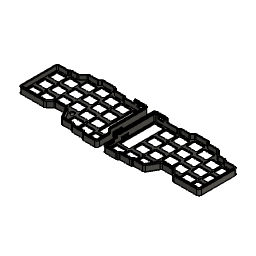
mriya-bumper-sla-v1.0.0 (Autodesk Fusion 360 design; units mm, degrees)
Autodesk Fusion 360 part; units mm, degrees
note: some values were not read from the file. Set by a fixed rule: which sketch regions a step uses.
(part 1 of 2)
sketch "mriya" plane through (0, 0, 0) normal (0, 0, 1) x (1, 0, 0)
  line L0 (-96.0213, 15.6719) -> (-89.7787, 21.9145) construction
  line L1 (-21.4858, 1.079) -> (-22.6142, 2.2074) construction
  line L2 (-133.1, 14.7932) -> (-98.1426, 14.7932) construction
  line L3 (-39.0716, 2.7932) -> (-24.0284, 2.7932) construction
  line L4 (-3.6, 0.4932) -> (-20.0716, 0.4932) construction
  line L5 (-59.4741, 6.1094) -> (-67.7517, 20.7608) construction
  line L6 (-40.4858, 3.379) -> (-41.6142, 4.5074) construction
  line L7 (-117.6142, 71.579) -> (-116.4858, 72.7074) construction
  line L8 (-96.0716, 81.2932) -> (-82.2284, 81.2932) construction
  line L9 (-133.1, 70.9932) -> (-119.0284, 70.9932) construction
  line L10 (-87.6574, 22.7932) -> (-71.2344, 22.7932) construction
  line L11 (-43.0284, 5.0932) -> (-57.7328, 5.0932) construction
  line L12 (-77.0716, 84.7932) -> (-59.7284, 84.7932) construction
  line L13 (-53.5716, 80.2932) -> (-40.7284, 80.2932) construction
  line L14 (-19.1, 19.4932) -> (-2.1, 19.4932) construction
  line L15 (-20.6, 20.9932) -> (-20.6, 77.9932) construction
  line L16 (-78.4858, 84.2074) -> (-80.8142, 81.879) construction
  line L17 (-58.3142, 84.2074) -> (-54.9858, 80.879) construction
  line L18 (-134.6, 69.4932) -> (-134.6, 16.2932) construction
  line L19 (-38.1858, 78.579) -> (-39.3142, 79.7074) construction
  line L20 (-94.4, 40.3932) -> (-94.4, 27.9932) construction
  line L21 (-93.6, 41.1932) -> (-81.2, 41.1932) construction
  line L22 (-93.6, 27.1932) -> (-81.2, 27.1932) construction
  line L23 (-80.4, 40.3932) -> (-80.4, 27.9932) construction
  line L24 (-37.4, 56.0932) -> (-37.4, 43.6932) construction
  line L25 (-36.6, 56.8932) -> (-24.2, 56.8932) construction
  line L26 (-36.6, 42.8932) -> (-24.2, 42.8932) construction
  line L27 (-23.4, 56.0932) -> (-23.4, 43.6932) construction
  line L28 (-56.4, 58.3932) -> (-56.4, 45.9932) construction
  line L29 (-55.6, 59.1932) -> (-43.2, 59.1932) construction
  line L30 (-55.6, 45.1932) -> (-43.2, 45.1932) construction
  line L31 (-42.4, 58.3932) -> (-42.4, 45.9932) construction
  line L32 (-132.4, 68.0932) -> (-132.4, 55.6932) construction
  line L33 (-131.6, 68.8932) -> (-119.2, 68.8932) construction
  line L34 (-131.6, 54.8932) -> (-119.2, 54.8932) construction
  line L35 (-118.4, 68.0932) -> (-118.4, 55.6932) construction
  line L36 (-56.4, 39.3932) -> (-56.4, 26.9932) construction
  line L37 (-55.6, 40.1932) -> (-43.2, 40.1932) construction
  line L38 (-55.6, 26.1932) -> (-43.2, 26.1932) construction
  line L39 (-42.4, 39.3932) -> (-42.4, 26.9932) construction
  line L40 (-37.4, 18.0932) -> (-37.4, 5.6932) construction
  line L41 (-36.6, 18.8932) -> (-24.2, 18.8932) construction
  line L42 (-36.6, 4.8932) -> (-24.2, 4.8932) construction
  line L43 (-23.4, 18.0932) -> (-23.4, 5.6932) construction
  line L44 (-18.4, 15.7932) -> (-18.4, 3.3932) construction
  line L45 (-17.6, 16.5932) -> (-5.2, 16.5932) construction
  line L46 (-17.6, 2.5932) -> (-5.2, 2.5932) construction
  line L47 (-4.4, 15.7932) -> (-4.4, 3.3932) construction
  line L48 (-132.4, 49.0932) -> (-132.4, 36.6932) construction
  line L49 (-131.6, 49.8932) -> (-119.2, 49.8932) construction
  line L50 (-131.6, 35.8932) -> (-119.2, 35.8932) construction
  line L51 (-118.4, 49.0932) -> (-118.4, 36.6932) construction
  line L52 (-113.4, 51.3932) -> (-113.4, 38.9932) construction
  line L53 (-112.6, 52.1932) -> (-100.2, 52.1932) construction
  line L54 (-112.6, 38.1932) -> (-100.2, 38.1932) construction
  line L55 (-99.4, 51.3932) -> (-99.4, 38.9932) construction
  line L56 (-132.4, 30.0932) -> (-132.4, 17.6932) construction
  line L57 (-131.6, 30.8932) -> (-119.2, 30.8932) construction
  line L58 (-131.6, 16.8932) -> (-119.2, 16.8932) construction
  line L59 (-118.4, 30.0932) -> (-118.4, 17.6932) construction
  line L60 (-56.4, 20.3932) -> (-56.4, 7.9932) construction
  line L61 (-55.6, 21.1932) -> (-43.2, 21.1932) construction
  line L62 (-55.6, 7.1932) -> (-43.2, 7.1932) construction
  line L63 (-42.4, 20.3932) -> (-42.4, 7.9932) construction
  line L64 (-75.4, 43.8932) -> (-75.4, 31.4932) construction
  line L65 (-74.6, 44.6932) -> (-62.2, 44.6932) construction
  line L66 (-74.6, 30.6932) -> (-62.2, 30.6932) construction
  line L67 (-61.4, 43.8932) -> (-61.4, 31.4932) construction
  line L68 (-75.4, 81.8932) -> (-75.4, 69.4932) construction
  line L69 (-74.6, 82.6932) -> (-62.2, 82.6932) construction
  line L70 (-74.6, 68.6932) -> (-62.2, 68.6932) construction
  line L71 (-61.4, 81.8932) -> (-61.4, 69.4932) construction
  line L72 (-37.4, 37.0932) -> (-37.4, 24.6932) construction
  line L73 (-36.6, 37.8932) -> (-24.2, 37.8932) construction
  line L74 (-36.6, 23.8932) -> (-24.2, 23.8932) construction
  line L75 (-23.4, 37.0932) -> (-23.4, 24.6932) construction
  line L76 (-113.4, 32.3932) -> (-113.4, 19.9932) construction
  line L77 (-112.6, 33.1932) -> (-100.2, 33.1932) construction
  line L78 (-112.6, 19.1932) -> (-100.2, 19.1932) construction
  line L79 (-99.4, 32.3932) -> (-99.4, 19.9932) construction
  line L80 (-56.4, 77.3932) -> (-56.4, 64.9932) construction
  line L81 (-55.6, 78.1932) -> (-43.2, 78.1932) construction
  line L82 (-55.6, 64.1932) -> (-43.2, 64.1932) construction
  line L83 (-42.4, 77.3932) -> (-42.4, 64.9932) construction
  line L84 (-37.4, 75.0932) -> (-37.4, 62.6932) construction
  line L85 (-36.6, 75.8932) -> (-24.2, 75.8932) construction
  line L86 (-36.6, 61.8932) -> (-24.2, 61.8932) construction
  line L87 (-23.4, 75.0932) -> (-23.4, 62.6932) construction
  line L88 (-113.4, 70.3932) -> (-113.4, 57.9932) construction
  line L89 (-112.6, 71.1932) -> (-100.2, 71.1932) construction
  line L90 (-112.6, 57.1932) -> (-100.2, 57.1932) construction
  line L91 (-99.4, 70.3932) -> (-99.4, 57.9932) construction
  line L92 (-94.4, 59.3932) -> (-94.4, 46.9932) construction
  line L93 (-93.6, 60.1932) -> (-81.2, 60.1932) construction
  line L94 (-93.6, 46.1932) -> (-81.2, 46.1932) construction
  line L95 (-80.4, 59.3932) -> (-80.4, 46.9932) construction
  line L96 (-75.4, 62.8932) -> (-75.4, 50.4932) construction
  line L97 (-74.6, 63.6932) -> (-62.2, 63.6932) construction
  line L98 (-74.6, 49.6932) -> (-62.2, 49.6932) construction
  line L99 (-61.4, 62.8932) -> (-61.4, 50.4932) construction
  line L100 (-94.4, 78.3932) -> (-94.4, 65.9932) construction
  line L101 (-93.6, 79.1932) -> (-81.2, 79.1932) construction
  line L102 (-93.6, 65.1932) -> (-81.2, 65.1932) construction
  line L103 (-80.4, 78.3932) -> (-80.4, 65.9932) construction
  circle A0 centre (-115.9, 53.5432) radius 1.6
  circle A1 centre (-115.9, 34.5432) radius 1.6
  circle A2 centre (-63.5, 23.5932) radius 3.5
  circle A3 centre (-39.9, 22.5432) radius 1.6
  circle A4 centre (-39.9, 60.5432) radius 1.6
  arc A5 (-38.1858, 78.579) -> (-36.7716, 77.9932) centre (-36.7716, 79.9932) ccw construction
  arc A6 (-39.3142, 79.7074) -> (-40.7284, 80.2932) centre (-40.7285, 78.2931) ccw construction
  arc A7 (-54.9858, 80.879) -> (-53.5716, 80.2932) centre (-53.5716, 82.2931) ccw construction
  arc A8 (-58.3142, 84.2074) -> (-59.7284, 84.7932) centre (-59.7285, 82.7931) ccw construction
  arc A9 (-77.0716, 84.7932) -> (-78.4858, 84.2074) centre (-77.0716, 82.7933) ccw construction
  arc A10 (-82.2284, 81.2932) -> (-80.8142, 81.879) centre (-82.2284, 83.2932) ccw construction
  arc A11 (-96.0716, 81.2932) -> (-97.4858, 80.7074) centre (-96.0716, 79.2933) ccw construction
  arc A12 (-115.0716, 73.2932) -> (-116.4858, 72.7074) centre (-115.0716, 71.2933) ccw construction
  arc A13 (-119.0284, 70.9932) -> (-117.6142, 71.579) centre (-119.0284, 72.9932) ccw construction
  arc A14 (-133.1, 70.9932) -> (-134.6, 69.4932) centre (-133.1, 69.4932) ccw construction
  arc A15 (-134.6, 16.2932) -> (-133.1, 14.7932) centre (-133.1, 16.2932) ccw construction
  arc A16 (-98.1426, 14.7932) -> (-96.0213, 15.6719) centre (-98.1426, 17.7931) ccw construction
  arc A17 (-87.6574, 22.7932) -> (-89.7787, 21.9145) centre (-87.6573, 19.7931) ccw construction
  arc A18 (-67.7517, 20.7608) -> (-71.2344, 22.7932) centre (-71.2344, 18.793) ccw construction
  arc A19 (-59.4741, 6.1094) -> (-57.7328, 5.0932) centre (-57.7328, 7.0932) ccw construction
  arc A20 (-41.6142, 4.5074) -> (-43.0284, 5.0932) centre (-43.0284, 3.0933) ccw construction
  arc A21 (-40.4858, 3.379) -> (-39.0716, 2.7932) centre (-39.0715, 4.7933) ccw construction
  arc A22 (-22.6142, 2.2074) -> (-24.0284, 2.7932) centre (-24.0284, 0.7933) ccw construction
  arc A23 (-21.4858, 1.079) -> (-20.0716, 0.4932) centre (-20.0715, 2.4933) ccw construction
  arc A24 (-3.6, 0.4932) -> (-2.1, 1.9932) centre (-3.6, 1.9932) ccw construction
  arc A25 (-20.6, 20.9932) -> (-19.1, 19.4932) centre (-19.1, 20.9932) ccw construction
  line L104 (-2.1, 1.9932) -> (-2.1, 76.4932) construction
  line L105 (-36.7716, 77.9932) -> (-3.6, 77.9932) construction
  arc A26 (-2.1, 76.4932) -> (-3.6, 77.9932) centre (-3.6, 76.4932) ccw construction
  arc A27 (-131.6, 68.8932) -> (-132.4, 68.0932) centre (-131.6, 68.0932) ccw construction
  arc A28 (-118.4, 68.0932) -> (-119.2, 68.8932) centre (-119.2, 68.0932) ccw construction
  arc A29 (-119.2, 54.8932) -> (-118.4, 55.6932) centre (-119.2, 55.6932) ccw construction
  arc A30 (-132.4, 55.6932) -> (-131.6, 54.8932) centre (-131.6, 55.6932) ccw construction
  arc A31 (-131.6, 49.8932) -> (-132.4, 49.0932) centre (-131.6, 49.0932) ccw construction
  arc A32 (-118.4, 49.0932) -> (-119.2, 49.8932) centre (-119.2, 49.0932) ccw construction
  arc A33 (-119.2, 35.8932) -> (-118.4, 36.6932) centre (-119.2, 36.6932) ccw construction
  arc A34 (-132.4, 36.6932) -> (-131.6, 35.8932) centre (-131.6, 36.6932) ccw construction
  arc A35 (-131.6, 30.8932) -> (-132.4, 30.0932) centre (-131.6, 30.0932) ccw construction
  arc A36 (-118.4, 30.0932) -> (-119.2, 30.8932) centre (-119.2, 30.0932) ccw construction
  arc A37 (-119.2, 16.8932) -> (-118.4, 17.6932) centre (-119.2, 17.6932) ccw construction
  arc A38 (-132.4, 17.6932) -> (-131.6, 16.8932) centre (-131.6, 17.6932) ccw construction
  arc A39 (-113.4, 19.9932) -> (-112.6, 19.1932) centre (-112.6, 19.9932) ccw construction
  arc A40 (-100.2, 19.1932) -> (-99.4, 19.9932) centre (-100.2, 19.9932) ccw construction
  arc A41 (-99.4, 32.3932) -> (-100.2, 33.1932) centre (-100.2, 32.3932) ccw construction
  arc A42 (-112.6, 33.1932) -> (-113.4, 32.3932) centre (-112.6, 32.3932) ccw construction
  arc A43 (-100.2, 38.1932) -> (-99.4, 38.9932) centre (-100.2, 38.9932) ccw construction
  arc A44 (-113.4, 38.9932) -> (-112.6, 38.1932) centre (-112.6, 38.9932) ccw construction
  arc A45 (-112.6, 52.1932) -> (-113.4, 51.3932) centre (-112.6, 51.3932) ccw construction
  arc A46 (-99.4, 51.3932) -> (-100.2, 52.1932) centre (-100.2, 51.3932) ccw construction
  arc A47 (-113.4, 57.9932) -> (-112.6, 57.1932) centre (-112.6, 57.9932) ccw construction
  arc A48 (-100.2, 57.1932) -> (-99.4, 57.9932) centre (-100.2, 57.9932) ccw construction
  arc A49 (-99.4, 70.3932) -> (-100.2, 71.1932) centre (-100.2, 70.3932) ccw construction
  arc A50 (-112.6, 71.1932) -> (-113.4, 70.3932) centre (-112.6, 70.3932) ccw construction
  arc A51 (-93.6, 79.1932) -> (-94.4, 78.3932) centre (-93.6, 78.3932) ccw construction
  arc A52 (-80.4, 78.3932) -> (-81.2, 79.1932) centre (-81.2, 78.3932) ccw construction
  arc A53 (-81.2, 65.1932) -> (-80.4, 65.9932) centre (-81.2, 65.9932) ccw construction
  arc A54 (-94.4, 65.9932) -> (-93.6, 65.1932) centre (-93.6, 65.9932) ccw construction
  arc A55 (-93.6, 60.1932) -> (-94.4, 59.3932) centre (-93.6, 59.3932) ccw construction
  arc A56 (-80.4, 59.3932) -> (-81.2, 60.1932) centre (-81.2, 59.3932) ccw construction
  arc A57 (-81.2, 46.1932) -> (-80.4, 46.9932) centre (-81.2, 46.9932) ccw construction
  arc A58 (-94.4, 46.9932) -> (-93.6, 46.1932) centre (-93.6, 46.9932) ccw construction
  arc A59 (-93.6, 41.1932) -> (-94.4, 40.3932) centre (-93.6, 40.3932) ccw construction
  arc A60 (-94.4, 27.9932) -> (-93.6, 27.1932) centre (-93.6, 27.9932) ccw construction
  arc A61 (-81.2, 27.1932) -> (-80.4, 27.9932) centre (-81.2, 27.9932) ccw construction
  arc A62 (-80.4, 40.3932) -> (-81.2, 41.1932) centre (-81.2, 40.3932) ccw construction
  arc A63 (-75.4, 31.4932) -> (-74.6, 30.6932) centre (-74.6, 31.4932) ccw construction
  arc A64 (-74.6, 44.6932) -> (-75.4, 43.8932) centre (-74.6, 43.8932) ccw construction
  arc A65 (-61.4, 43.8932) -> (-62.2, 44.6932) centre (-62.2, 43.8932) ccw construction
  arc A66 (-62.2, 30.6932) -> (-61.4, 31.4932) centre (-62.2, 31.4932) ccw construction
  arc A67 (-62.2, 49.6932) -> (-61.4, 50.4932) centre (-62.2, 50.4932) ccw construction
  arc A68 (-75.4, 50.4932) -> (-74.6, 49.6932) centre (-74.6, 50.4932) ccw construction
  arc A69 (-74.6, 63.6932) -> (-75.4, 62.8932) centre (-74.6, 62.8932) ccw construction
  arc A70 (-61.4, 62.8932) -> (-62.2, 63.6932) centre (-62.2, 62.8932) ccw construction
  arc A71 (-62.2, 68.6932) -> (-61.4, 69.4932) centre (-62.2, 69.4932) ccw construction
  arc A72 (-75.4, 69.4932) -> (-74.6, 68.6932) centre (-74.6, 69.4932) ccw construction
  arc A73 (-74.6, 82.6932) -> (-75.4, 81.8932) centre (-74.6, 81.8932) ccw construction
  arc A74 (-61.4, 81.8932) -> (-62.2, 82.6932) centre (-62.2, 81.8932) ccw construction
  arc A75 (-55.6, 78.1932) -> (-56.4, 77.3932) centre (-55.6, 77.3932) ccw construction
  arc A76 (-56.4, 64.9932) -> (-55.6, 64.1932) centre (-55.6, 64.9932) ccw construction
  arc A77 (-43.2, 64.1932) -> (-42.4, 64.9932) centre (-43.2, 64.9932) ccw construction
  arc A78 (-42.4, 77.3932) -> (-43.2, 78.1932) centre (-43.2, 77.3932) ccw construction
  arc A79 (-42.4, 58.3932) -> (-43.2, 59.1932) centre (-43.2, 58.3932) ccw construction
  arc A80 (-55.6, 59.1932) -> (-56.4, 58.3932) centre (-55.6, 58.3932) ccw construction
  arc A81 (-56.4, 45.9932) -> (-55.6, 45.1932) centre (-55.6, 45.9932) ccw construction
  arc A82 (-43.2, 45.1932) -> (-42.4, 45.9932) centre (-43.2, 45.9932) ccw construction
  arc A83 (-42.4, 39.3932) -> (-43.2, 40.1932) centre (-43.2, 39.3932) ccw construction
  arc A84 (-55.6, 40.1932) -> (-56.4, 39.3932) centre (-55.6, 39.3932) ccw construction
  arc A85 (-56.4, 26.9932) -> (-55.6, 26.1932) centre (-55.6, 26.9932) ccw construction
  arc A86 (-43.2, 26.1932) -> (-42.4, 26.9932) centre (-43.2, 26.9932) ccw construction
  arc A87 (-42.4, 20.3932) -> (-43.2, 21.1932) centre (-43.2, 20.3932) ccw construction
  arc A88 (-55.6, 21.1932) -> (-56.4, 20.3932) centre (-55.6, 20.3932) ccw construction
  arc A89 (-56.4, 7.9932) -> (-55.6, 7.1932) centre (-55.6, 7.9932) ccw construction
  arc A90 (-43.2, 7.1932) -> (-42.4, 7.9932) centre (-43.2, 7.9932) ccw construction
  arc A91 (-37.4, 5.6932) -> (-36.6, 4.8932) centre (-36.6, 5.6932) ccw construction
  arc A92 (-24.2, 4.8932) -> (-23.4, 5.6932) centre (-24.2, 5.6932) ccw construction
  arc A93 (-23.4, 18.0932) -> (-24.2, 18.8932) centre (-24.2, 18.0932) ccw construction
  arc A94 (-36.6, 18.8932) -> (-37.4, 18.0932) centre (-36.6, 18.0932) ccw construction
  arc A95 (-18.4, 3.3932) -> (-17.6, 2.5932) centre (-17.6, 3.3932) ccw construction
  arc A96 (-5.2, 2.5932) -> (-4.4, 3.3932) centre (-5.2, 3.3932) ccw construction
  arc A97 (-4.4, 15.7932) -> (-5.2, 16.5932) centre (-5.2, 15.7932) ccw construction
  arc A98 (-17.6, 16.5932) -> (-18.4, 15.7932) centre (-17.6, 15.7932) ccw construction
  arc A99 (-24.2, 23.8932) -> (-23.4, 24.6932) centre (-24.2, 24.6932) ccw construction
  arc A100 (-37.4, 24.6932) -> (-36.6, 23.8932) centre (-36.6, 24.6932) ccw construction
  arc A101 (-36.6, 37.8932) -> (-37.4, 37.0932) centre (-36.6, 37.0932) ccw construction
  arc A102 (-23.4, 37.0932) -> (-24.2, 37.8932) centre (-24.2, 37.0932) ccw construction
  arc A103 (-24.2, 42.8932) -> (-23.4, 43.6932) centre (-24.2, 43.6932) ccw construction
  arc A104 (-37.4, 43.6932) -> (-36.6, 42.8932) centre (-36.6, 43.6932) ccw construction
  arc A105 (-36.6, 56.8932) -> (-37.4, 56.0932) centre (-36.6, 56.0932) ccw construction
  arc A106 (-23.4, 56.0932) -> (-24.2, 56.8932) centre (-24.2, 56.0932) ccw construction
  arc A107 (-24.2, 61.8932) -> (-23.4, 62.6932) centre (-24.2, 62.6932) ccw construction
  arc A108 (-37.4, 62.6932) -> (-36.6, 61.8932) centre (-36.6, 62.6932) ccw construction
  arc A109 (-36.6, 75.8932) -> (-37.4, 75.0932) centre (-36.6, 75.0932) ccw construction
  arc A110 (-23.4, 75.0932) -> (-24.2, 75.8932) centre (-24.2, 75.0932) ccw construction
  line L106 (-117.6496, 71.6144) -> (-116.5212, 72.7428)
  arc A111 (-115.0716, 73.3432) -> (-116.5212, 72.7428) centre (-115.0716, 71.2933) ccw
  arc A112 (-96.0716, 81.3432) -> (-97.5212, 80.7428) centre (-96.0716, 79.2933) ccw
  line L107 (-96.0716, 81.3432) -> (-82.2284, 81.3432)
  arc A113 (-82.2284, 81.3432) -> (-80.8496, 81.9144) centre (-82.2284, 83.2932) ccw
  line L108 (-78.5212, 84.2428) -> (-80.8496, 81.9144)
  arc A114 (-77.0716, 84.8432) -> (-78.5212, 84.2428) centre (-77.0716, 82.7933) ccw
  line L109 (-77.0716, 84.8432) -> (-59.7284, 84.8432)
  arc A115 (-58.2788, 84.2427) -> (-59.7284, 84.8432) centre (-59.7285, 82.7931) ccw
  line L110 (-58.2788, 84.2427) -> (-54.9504, 80.9144)
  arc A116 (-54.9504, 80.9144) -> (-53.5716, 80.3432) centre (-53.5716, 82.2931) ccw
  line L111 (-53.5716, 80.3432) -> (-40.7284, 80.3432)
  arc A117 (-39.2788, 79.7427) -> (-40.7284, 80.3432) centre (-40.7285, 78.2931) ccw
  line L112 (-38.1504, 78.6144) -> (-39.2788, 79.7427)
  arc A118 (-38.1504, 78.6144) -> (-36.7716, 78.0432) centre (-36.7716, 79.9932) ccw
  line L113 (-36.7716, 78.0432) -> (-3.6, 78.0432)
  arc A119 (-2.05, 76.4932) -> (-3.6, 78.0432) centre (-3.6, 76.4932) ccw
  line L114 (-2.05, 1.9932) -> (-2.05, 76.4932)
  arc A120 (-3.6, 0.4432) -> (-2.05, 1.9932) centre (-3.6, 1.9932) ccw
  line L115 (-3.6, 0.4432) -> (-20.0716, 0.4432)
  arc A121 (-21.5212, 1.0437) -> (-20.0716, 0.4432) centre (-20.0715, 2.4933) ccw
  line L116 (-21.5212, 1.0437) -> (-22.6496, 2.172)
  arc A122 (-22.6496, 2.172) -> (-24.0284, 2.7432) centre (-24.0284, 0.7933) ccw
  line L117 (-39.0716, 2.7432) -> (-24.0284, 2.7432)
  arc A123 (-40.5212, 3.3437) -> (-39.0716, 2.7432) centre (-39.0715, 4.7933) ccw
  line L118 (-40.5212, 3.3437) -> (-41.6496, 4.472)
  arc A124 (-41.6496, 4.472) -> (-43.0284, 5.0432) centre (-43.0284, 3.0933) ccw
  line L119 (-43.0284, 5.0432) -> (-57.7328, 5.0432)
  arc A125 (-59.5176, 6.0848) -> (-57.7328, 5.0432) centre (-57.7328, 7.0932) ccw
  line L120 (-59.5176, 6.0848) -> (-67.7952, 20.7362)
  arc A126 (-67.7952, 20.7362) -> (-71.2344, 22.7432) centre (-71.2344, 18.793) ccw
  line L121 (-87.6574, 22.7432) -> (-71.2344, 22.7432)
  arc A127 (-87.6574, 22.7432) -> (-89.7433, 21.8791) centre (-87.6573, 19.7931) ccw
  line L122 (-95.9859, 15.6365) -> (-89.7433, 21.8791)
  arc A128 (-98.1426, 14.7432) -> (-95.9859, 15.6365) centre (-98.1426, 17.7931) ccw
  line L123 (-133.1, 14.7432) -> (-98.1426, 14.7432)
  arc A129 (-134.65, 16.2932) -> (-133.1, 14.7432) centre (-133.1, 16.2932) ccw
  line L124 (-134.65, 69.4932) -> (-134.65, 16.2932)
  arc A130 (-133.1, 71.0432) -> (-134.65, 69.4932) centre (-133.1, 69.4932) ccw
  line L125 (-133.1, 71.0432) -> (-119.0284, 71.0432)
  arc A131 (-119.0284, 71.0432) -> (-117.6496, 71.6144) centre (-119.0284, 72.9932) ccw
  line L126 (-77.7136, 87.3432) -> (-59.0864, 87.3432)
  arc A132 (0.45, 76.4932) -> (-3.6, 80.5432) centre (-3.6, 76.4932) ccw
  line L127 (0.45, 1.9932) -> (0.45, 76.4932)
  arc A133 (-3.6, -2.0568) -> (0.45, 1.9932) centre (-3.6, 1.9932) ccw
  line L128 (-3.6, -2.0568) -> (-20.7136, -2.0568)
  line L129 (-133.1, 12.2432) -> (-97.7077, 12.2432)
  arc A134 (-137.15, 16.2932) -> (-133.1, 12.2432) centre (-133.1, 16.2932) ccw
  line L130 (-137.15, 69.4932) -> (-137.15, 16.2932)
  arc A135 (-133.1, 73.5432) -> (-137.15, 69.4932) centre (-133.1, 69.4932) ccw
  circle A136 centre (-17.6, 22.4932) radius 1.1 construction
  circle A137 centre (-5.2, 22.4932) radius 1.1 construction
  line L131 (-2.05, 19.1932) -> (0.45, 19.1932)
  line L132 (-20.9, 78.0432) -> (-20.9, 80.5432)
  line L133 (-19.7, 77.8432) -> (-19.7, 78.0432)
  line L134 (-19.1, 77.2432) -> (-3.65, 77.2432)
  line L135 (-2.25, 21.1932) -> (-2.05, 21.1932)
  line L136 (-2.85, 21.7932) -> (-2.85, 76.4432)
  arc A138 (-2.85, 76.4432) -> (-3.65, 77.2432) centre (-3.65, 76.4432) ccw
  arc A139 (-19.7, 77.8432) -> (-19.1, 77.2432) centre (-19.1, 77.8432) ccw
  arc A140 (-2.85, 21.7932) -> (-2.25, 21.1932) centre (-2.25, 21.7932) ccw
  line L137 (-2.05, 14.5932) -> (-2.25, 14.5932)
  line L138 (-2.85, 13.9932) -> (-2.85, 5.1932)
  line L139 (-2.25, 4.5932) -> (-2.05, 4.5932)
  arc A141 (-2.25, 14.5932) -> (-2.85, 13.9932) centre (-2.25, 13.9932) ccw
  arc A142 (-2.85, 5.1932) -> (-2.25, 4.5932) centre (-2.25, 5.1932) ccw
  line L140 (-97.4858, 80.7074) -> (-104.0213, 74.1719) construction
  line L141 (-115.0716, 73.2932) -> (-106.1426, 73.2932) construction
  line L142 (-97.5212, 80.7428) -> (-104.0567, 74.2072)
  line L143 (-106.1426, 73.3432) -> (-115.0716, 73.3432)
  arc A143 (-106.1426, 73.3432) -> (-104.0567, 74.2072) centre (-106.1426, 76.2932) ccw
  arc A144 (-106.1426, 73.2932) -> (-104.0213, 74.1719) centre (-106.1426, 76.2932) ccw construction
  line L144 (-87.0153, 20.2432) -> (-72.1389, 20.2432)
  arc A145 (-87.0153, 20.2432) -> (-88.4295, 19.6574) centre (-87.0153, 18.2432) ccw
  arc A146 (-69.5269, 18.7189) -> (-72.1389, 20.2432) centre (-72.1389, 17.2432) ccw
  line L145 (-106.3705, 75.8432) -> (-115.7136, 75.8432)
  line L146 (-133.1, 73.5432) -> (-119.6705, 73.5432)
  line L147 (-96.7136, 83.8432) -> (-82.8705, 83.8432)
  line L148 (-52.9295, 82.8432) -> (-40.0864, 82.8432)
  line L149 (-36.1295, 80.5432) -> (-3.6, 80.5432)
  line L150 (-39.7136, 0.2432) -> (-24.6705, 0.2432)
  line L151 (-58.3456, 2.5432) -> (-43.6705, 2.5432)
  arc A147 (-59.7284, 82.7932) -> (-59.7285, 82.7932) centre (-59.7285, 82.7931) ccw
  arc A148 (-40.7284, 78.2932) -> (-40.7285, 78.2932) centre (-40.7285, 78.2931) ccw
  arc A149 (-20.0716, 2.4932) -> (-20.0715, 2.4932) centre (-20.0715, 2.4933) ccw
  arc A150 (-39.0716, 4.7932) -> (-39.0715, 4.7932) centre (-39.0715, 4.7933) ccw
  line L152 (-118.9, 54.8932) -> (-131.9, 54.8932)
  line L153 (-133.9, 56.8932) -> (-133.9, 66.8932)
  line L154 (-131.9, 68.8932) -> (-118.9, 68.8932)
  line L155 (-116.9, 66.8932) -> (-116.9, 56.8932)
  arc A151 (-116.9, 66.8932) -> (-118.9, 68.8932) centre (-118.9, 66.8932) ccw
  arc A152 (-118.9, 54.8932) -> (-116.9, 56.8932) centre (-118.9, 56.8932) ccw
  arc A153 (-133.9, 56.8932) -> (-131.9, 54.8932) centre (-131.9, 56.8932) ccw
  arc A154 (-131.9, 68.8932) -> (-133.9, 66.8932) centre (-131.9, 66.8932) ccw
  arc A155 (-118.9, 35.8932) -> (-116.9, 37.8932) centre (-118.9, 37.8932) ccw
  line L156 (-118.9, 35.8932) -> (-131.9, 35.8932)
  arc A156 (-133.9, 37.8932) -> (-131.9, 35.8932) centre (-131.9, 37.8932) ccw
  line L157 (-133.9, 37.8932) -> (-133.9, 47.8932)
  arc A157 (-131.9, 49.8932) -> (-133.9, 47.8932) centre (-131.9, 47.8932) ccw
  line L158 (-131.9, 49.8932) -> (-118.9, 49.8932)
  arc A158 (-116.9, 47.8932) -> (-118.9, 49.8932) centre (-118.9, 47.8932) ccw
  line L159 (-116.9, 47.8932) -> (-116.9, 37.8932)
  arc A159 (-118.9, 16.8932) -> (-116.9, 18.8932) centre (-118.9, 18.8932) ccw
  line L160 (-118.9, 16.8932) -> (-131.9, 16.8932)
  arc A160 (-133.9, 18.8932) -> (-131.9, 16.8932) centre (-131.9, 18.8932) ccw
  line L161 (-133.9, 18.8932) -> (-133.9, 28.8932)
  arc A161 (-131.9, 30.8932) -> (-133.9, 28.8932) centre (-131.9, 28.8932) ccw
  line L162 (-131.9, 30.8932) -> (-118.9, 30.8932)
  arc A162 (-116.9, 28.8932) -> (-118.9, 30.8932) centre (-118.9, 28.8932) ccw
  line L163 (-116.9, 28.8932) -> (-116.9, 18.8932)
  arc A163 (-99.9, 57.1932) -> (-97.9, 59.1932) centre (-99.9, 59.1932) ccw
  line L164 (-99.9, 57.1932) -> (-112.9, 57.1932)
  arc A164 (-114.9, 59.1932) -> (-112.9, 57.1932) centre (-112.9, 59.1932) ccw
  line L165 (-114.9, 59.1932) -> (-114.9, 69.1932)
  arc A165 (-112.9, 71.1932) -> (-114.9, 69.1932) centre (-112.9, 69.1932) ccw
  line L166 (-112.9, 71.1932) -> (-99.9, 71.1932)
  arc A166 (-97.9, 69.1932) -> (-99.9, 71.1932) centre (-99.9, 69.1932) ccw
  line L167 (-97.9, 69.1932) -> (-97.9, 59.1932)
  arc A167 (-99.9, 38.1932) -> (-97.9, 40.1932) centre (-99.9, 40.1932) ccw
  line L168 (-99.9, 38.1932) -> (-112.9, 38.1932)
  arc A168 (-114.9, 40.1932) -> (-112.9, 38.1932) centre (-112.9, 40.1932) ccw
  line L169 (-114.9, 40.1932) -> (-114.9, 50.1932)
  arc A169 (-112.9, 52.1932) -> (-114.9, 50.1932) centre (-112.9, 50.1932) ccw
  line L170 (-112.9, 52.1932) -> (-99.9, 52.1932)
  arc A170 (-97.9, 50.1932) -> (-99.9, 52.1932) centre (-99.9, 50.1932) ccw
  line L171 (-97.9, 50.1932) -> (-97.9, 40.1932)
  arc A171 (-99.9, 19.1932) -> (-97.9, 21.1932) centre (-99.9, 21.1932) ccw
  line L172 (-99.9, 19.1932) -> (-112.9, 19.1932)
  arc A172 (-114.9, 21.1932) -> (-112.9, 19.1932) centre (-112.9, 21.1932) ccw
  line L173 (-114.9, 21.1932) -> (-114.9, 31.1932)
  arc A173 (-112.9, 33.1932) -> (-114.9, 31.1932) centre (-112.9, 31.1932) ccw
  line L174 (-112.9, 33.1932) -> (-99.9, 33.1932)
  arc A174 (-97.9, 31.1932) -> (-99.9, 33.1932) centre (-99.9, 31.1932) ccw
  line L175 (-97.9, 31.1932) -> (-97.9, 21.1932)
  arc A175 (-80.9, 65.1932) -> (-78.9, 67.1932) centre (-80.9, 67.1932) ccw
  line L176 (-80.9, 65.1932) -> (-93.9, 65.1932)
  arc A176 (-95.9, 67.1932) -> (-93.9, 65.1932) centre (-93.9, 67.1932) ccw
  line L177 (-95.9, 67.1932) -> (-95.9, 77.1932)
  arc A177 (-93.9, 79.1932) -> (-95.9, 77.1932) centre (-93.9, 77.1932) ccw
  line L178 (-93.9, 79.1932) -> (-80.9, 79.1932)
  arc A178 (-78.9, 77.1932) -> (-80.9, 79.1932) centre (-80.9, 77.1932) ccw
  line L179 (-78.9, 77.1932) -> (-78.9, 67.1932)
  arc A179 (-80.9, 46.1932) -> (-78.9, 48.1932) centre (-80.9, 48.1932) ccw
  line L180 (-80.9, 46.1932) -> (-93.9, 46.1932)
  arc A180 (-95.9, 48.1932) -> (-93.9, 46.1932) centre (-93.9, 48.1932) ccw
  line L181 (-95.9, 48.1932) -> (-95.9, 58.1932)
  arc A181 (-93.9, 60.1932) -> (-95.9, 58.1932) centre (-93.9, 58.1932) ccw
  line L182 (-93.9, 60.1932) -> (-80.9, 60.1932)
  arc A182 (-78.9, 58.1932) -> (-80.9, 60.1932) centre (-80.9, 58.1932) ccw
  line L183 (-78.9, 58.1932) -> (-78.9, 48.1932)
  arc A183 (-80.9, 27.1932) -> (-78.9, 29.1932) centre (-80.9, 29.1932) ccw
  line L184 (-80.9, 27.1932) -> (-93.9, 27.1932)
  arc A184 (-95.9, 29.1932) -> (-93.9, 27.1932) centre (-93.9, 29.1932) ccw
  line L185 (-95.9, 29.1932) -> (-95.9, 39.1932)
  arc A185 (-93.9, 41.1932) -> (-95.9, 39.1932) centre (-93.9, 39.1932) ccw
  line L186 (-93.9, 41.1932) -> (-80.9, 41.1932)
  arc A186 (-78.9, 39.1932) -> (-80.9, 41.1932) centre (-80.9, 39.1932) ccw
  line L187 (-78.9, 39.1932) -> (-78.9, 29.1932)
  arc A187 (-61.9, 30.6932) -> (-59.9, 32.6932) centre (-61.9, 32.6932) ccw
  line L188 (-61.9, 30.6932) -> (-74.9, 30.6932)
  arc A188 (-76.9, 32.6932) -> (-74.9, 30.6932) centre (-74.9, 32.6932) ccw
  line L189 (-76.9, 32.6932) -> (-76.9, 42.6932)
  arc A189 (-74.9, 44.6932) -> (-76.9, 42.6932) centre (-74.9, 42.6932) ccw
  line L190 (-74.9, 44.6932) -> (-61.9, 44.6932)
  arc A190 (-59.9, 42.6932) -> (-61.9, 44.6932) centre (-61.9, 42.6932) ccw
  line L191 (-59.9, 42.6932) -> (-59.9, 32.6932)
  arc A191 (-61.9, 49.6932) -> (-59.9, 51.6932) centre (-61.9, 51.6932) ccw
  line L192 (-61.9, 49.6932) -> (-74.9, 49.6932)
  arc A192 (-76.9, 51.6932) -> (-74.9, 49.6932) centre (-74.9, 51.6932) ccw
  line L193 (-76.9, 51.6932) -> (-76.9, 61.6932)
  arc A193 (-74.9, 63.6932) -> (-76.9, 61.6932) centre (-74.9, 61.6932) ccw
  line L194 (-74.9, 63.6932) -> (-61.9, 63.6932)
  arc A194 (-59.9, 61.6932) -> (-61.9, 63.6932) centre (-61.9, 61.6932) ccw
  line L195 (-59.9, 61.6932) -> (-59.9, 51.6932)
  arc A195 (-61.9, 68.6932) -> (-59.9, 70.6932) centre (-61.9, 70.6932) ccw
  line L196 (-61.9, 68.6932) -> (-74.9, 68.6932)
  arc A196 (-76.9, 70.6932) -> (-74.9, 68.6932) centre (-74.9, 70.6932) ccw
  line L197 (-76.9, 70.6932) -> (-76.9, 80.6932)
  arc A197 (-74.9, 82.6932) -> (-76.9, 80.6932) centre (-74.9, 80.6932) ccw
  line L198 (-74.9, 82.6932) -> (-61.9, 82.6932)
  arc A198 (-59.9, 80.6932) -> (-61.9, 82.6932) centre (-61.9, 80.6932) ccw
  line L199 (-59.9, 80.6932) -> (-59.9, 70.6932)
  arc A199 (-42.9, 26.1932) -> (-40.9, 28.1932) centre (-42.9, 28.1932) ccw
  line L200 (-42.9, 26.1932) -> (-55.9, 26.1932)
  arc A200 (-57.9, 28.1932) -> (-55.9, 26.1932) centre (-55.9, 28.1932) ccw
  line L201 (-57.9, 28.1932) -> (-57.9, 38.1932)
  arc A201 (-55.9, 40.1932) -> (-57.9, 38.1932) centre (-55.9, 38.1932) ccw
  line L202 (-55.9, 40.1932) -> (-42.9, 40.1932)
  arc A202 (-40.9, 38.1932) -> (-42.9, 40.1932) centre (-42.9, 38.1932) ccw
  line L203 (-40.9, 38.1932) -> (-40.9, 28.1932)
  arc A203 (-42.9, 45.1932) -> (-40.9, 47.1932) centre (-42.9, 47.1932) ccw
  line L204 (-42.9, 45.1932) -> (-55.9, 45.1932)
  arc A204 (-57.9, 47.1932) -> (-55.9, 45.1932) centre (-55.9, 47.1932) ccw
  line L205 (-57.9, 47.1932) -> (-57.9, 57.1932)
  arc A205 (-55.9, 59.1932) -> (-57.9, 57.1932) centre (-55.9, 57.1932) ccw
  line L206 (-55.9, 59.1932) -> (-42.9, 59.1932)
  arc A206 (-40.9, 57.1932) -> (-42.9, 59.1932) centre (-42.9, 57.1932) ccw
  line L207 (-40.9, 57.1932) -> (-40.9, 47.1932)
  arc A207 (-42.9, 64.1932) -> (-40.9, 66.1932) centre (-42.9, 66.1932) ccw
  line L208 (-42.9, 64.1932) -> (-55.9, 64.1932)
  arc A208 (-57.9, 66.1932) -> (-55.9, 64.1932) centre (-55.9, 66.1932) ccw
  line L209 (-57.9, 66.1932) -> (-57.9, 76.1932)
  arc A209 (-55.9, 78.1932) -> (-57.9, 76.1932) centre (-55.9, 76.1932) ccw
  line L210 (-55.9, 78.1932) -> (-42.9, 78.1932)
  arc A210 (-40.9, 76.1932) -> (-42.9, 78.1932) centre (-42.9, 76.1932) ccw
  line L211 (-40.9, 76.1932) -> (-40.9, 66.1932)
  arc A211 (-42.9, 7.1932) -> (-40.9, 9.1932) centre (-42.9, 9.1932) ccw
  line L212 (-42.9, 7.1932) -> (-55.9, 7.1932)
  arc A212 (-57.9, 9.1932) -> (-55.9, 7.1932) centre (-55.9, 9.1932) ccw
  line L213 (-57.9, 9.1932) -> (-57.9, 19.1932)
  arc A213 (-55.9, 21.1932) -> (-57.9, 19.1932) centre (-55.9, 19.1932) ccw
  line L214 (-55.9, 21.1932) -> (-42.9, 21.1932)
  arc A214 (-40.9, 19.1932) -> (-42.9, 21.1932) centre (-42.9, 19.1932) ccw
  line L215 (-40.9, 19.1932) -> (-40.9, 9.1932)
  arc A215 (-23.9, 4.8932) -> (-21.9, 6.8932) centre (-23.9, 6.8932) ccw
  line L216 (-23.9, 4.8932) -> (-36.9, 4.8932)
  arc A216 (-38.9, 6.8932) -> (-36.9, 4.8932) centre (-36.9, 6.8932) ccw
  line L217 (-38.9, 6.8932) -> (-38.9, 16.8932)
  arc A217 (-36.9, 18.8932) -> (-38.9, 16.8932) centre (-36.9, 16.8932) ccw
  line L218 (-36.9, 18.8932) -> (-23.9, 18.8932)
  arc A218 (-21.9, 16.8932) -> (-23.9, 18.8932) centre (-23.9, 16.8932) ccw
  line L219 (-21.9, 16.8932) -> (-21.9, 6.8932)
  arc A219 (-23.9, 23.8932) -> (-21.9, 25.8932) centre (-23.9, 25.8932) ccw
  line L220 (-23.9, 23.8932) -> (-36.9, 23.8932)
  arc A220 (-38.9, 25.8932) -> (-36.9, 23.8932) centre (-36.9, 25.8932) ccw
  line L221 (-38.9, 25.8932) -> (-38.9, 35.8932)
  arc A221 (-36.9, 37.8932) -> (-38.9, 35.8932) centre (-36.9, 35.8932) ccw
  line L222 (-36.9, 37.8932) -> (-23.9, 37.8932)
  arc A222 (-21.9, 35.8932) -> (-23.9, 37.8932) centre (-23.9, 35.8932) ccw
  line L223 (-21.9, 35.8932) -> (-21.9, 25.8932)
  arc A223 (-23.9, 42.8932) -> (-21.9, 44.8932) centre (-23.9, 44.8932) ccw
  line L224 (-23.9, 42.8932) -> (-36.9, 42.8932)
  arc A224 (-38.9, 44.8932) -> (-36.9, 42.8932) centre (-36.9, 44.8932) ccw
  line L225 (-38.9, 44.8932) -> (-38.9, 54.8932)
  arc A225 (-36.9, 56.8932) -> (-38.9, 54.8932) centre (-36.9, 54.8932) ccw
  line L226 (-36.9, 56.8932) -> (-23.9, 56.8932)
  arc A226 (-21.9, 54.8932) -> (-23.9, 56.8932) centre (-23.9, 54.8932) ccw
  line L227 (-21.9, 54.8932) -> (-21.9, 44.8932)
  arc A227 (-23.9, 61.8932) -> (-21.9, 63.8932) centre (-23.9, 63.8932) ccw
  line L228 (-23.9, 61.8932) -> (-36.9, 61.8932)
  arc A228 (-38.9, 63.8932) -> (-36.9, 61.8932) centre (-36.9, 63.8932) ccw
  line L229 (-38.9, 63.8932) -> (-38.9, 73.8932)
  arc A229 (-36.9, 75.8932) -> (-38.9, 73.8932) centre (-36.9, 73.8932) ccw
  line L230 (-36.9, 75.8932) -> (-23.9, 75.8932)
  arc A230 (-21.9, 73.8932) -> (-23.9, 75.8932) centre (-23.9, 73.8932) ccw
  line L231 (-21.9, 73.8932) -> (-21.9, 63.8932)
  arc A231 (-4.9, 2.5932) -> (-2.9, 4.5932) centre (-4.9, 4.5932) ccw
  line L232 (-4.9, 2.5932) -> (-17.9, 2.5932)
  arc A232 (-19.9, 4.5932) -> (-17.9, 2.5932) centre (-17.9, 4.5932) ccw
  line L233 (-19.9, 4.5932) -> (-19.9, 14.5932)
  arc A233 (-17.9, 16.5932) -> (-19.9, 14.5932) centre (-17.9, 14.5932) ccw
  line L234 (-17.9, 16.5932) -> (-4.9, 16.5932)
  arc A234 (-2.9, 14.5932) -> (-4.9, 16.5932) centre (-4.9, 14.5932) ccw
  line L235 (-2.9, 14.5932) -> (-2.9, 4.5932)
  arc A235 (-4.9, 19.8932) -> (-2.9, 21.8932) centre (-4.9, 21.8932) ccw
  line L236 (-4.9, 19.8932) -> (-17.9, 19.8932)
  arc A236 (-19.9, 21.8932) -> (-17.9, 19.8932) centre (-17.9, 21.8932) ccw
  line L237 (-19.9, 21.8932) -> (-19.9, 73.8932)
  arc A237 (-17.9, 75.8932) -> (-19.9, 73.8932) centre (-17.9, 73.8932) ccw
  line L238 (-17.9, 75.8932) -> (-4.9, 75.8932)
  arc A238 (-2.9, 73.8932) -> (-4.9, 75.8932) centre (-4.9, 73.8932) ccw
  line L239 (-2.9, 73.8932) -> (-2.9, 21.8932)
  arc A239 (-115.7136, 75.8432) -> (-117.8349, 74.9645) centre (-115.7136, 72.8432) ccw
  line L240 (-118.9634, 73.8361) -> (-117.8349, 74.9645)
  arc A240 (-119.6705, 73.5432) -> (-118.9634, 73.8361) centre (-119.6705, 74.5432) ccw
  line L241 (-105.6634, 76.1361) -> (-98.8349, 82.9645)
  arc A241 (-106.3705, 75.8432) -> (-105.6634, 76.1361) centre (-106.3705, 76.8432) ccw
  arc A242 (-96.7136, 83.8432) -> (-98.8349, 82.9645) centre (-96.7136, 80.8432) ccw
  line L242 (-82.1634, 84.1361) -> (-79.8349, 86.4645)
  arc A243 (-82.8705, 83.8432) -> (-82.1634, 84.1361) centre (-82.8705, 84.8432) ccw
  arc A244 (-77.7136, 87.3432) -> (-79.8349, 86.4645) centre (-77.7136, 84.3432) ccw
  line L243 (-53.6367, 83.1361) -> (-56.9651, 86.4645)
  arc A245 (-56.9651, 86.4645) -> (-59.0864, 87.3432) centre (-59.0864, 84.3432) ccw
  arc A246 (-53.6367, 83.1361) -> (-52.9295, 82.8432) centre (-52.9295, 83.8432) ccw
  line L244 (-36.8367, 80.8361) -> (-37.9651, 81.9645)
  arc A247 (-37.9651, 81.9645) -> (-40.0864, 82.8432) centre (-40.0864, 79.8432) ccw
  arc A248 (-36.8367, 80.8361) -> (-36.1295, 80.5432) centre (-36.1295, 81.5432) ccw
  line L245 (-42.9633, 2.2503) -> (-41.8349, 1.1219)
  arc A249 (-42.9633, 2.2503) -> (-43.6705, 2.5432) centre (-43.6705, 1.5432) ccw
  arc A250 (-41.8349, 1.1219) -> (-39.7136, 0.2432) centre (-39.7136, 3.2432) ccw
  line L246 (-69.5269, 18.7189) -> (-61.3929, 4.3216)
  arc A251 (-61.3929, 4.3216) -> (-58.3456, 2.5432) centre (-58.3456, 6.0432) ccw
  line L247 (-94.5257, 13.5612) -> (-88.4295, 19.6574)
  arc A252 (-97.7077, 12.2432) -> (-94.5257, 13.5612) centre (-97.7077, 16.7432) ccw
  line L248 (-23.9633, -0.0497) -> (-22.8349, -1.1781)
  arc A253 (-23.9633, -0.0497) -> (-24.6705, 0.2432) centre (-24.6705, -0.7568) ccw
  arc A254 (-22.8349, -1.1781) -> (-20.7136, -2.0568) centre (-20.7136, 0.9432) ccw
  dimension "d1" = 3.2
  dimension "d2" = 3.2
  dimension "d3" = 7
  dimension "d4" = 3.2
  dimension "d5" = 3.2
  dimension "d9" = 2.2
  dimension "d12" = 2.2
  constraint tangent L19 A5
  constraint tangent L19 A6
  constraint tangent L13 A7
  constraint tangent L17 A8
  constraint tangent L12 A9
  constraint tangent L16 A10
  constraint tangent L8 A11
  constraint tangent L7 A13
  constraint tangent L9 A14
  constraint tangent L18 A15
  constraint tangent L2 A16
  constraint tangent L0 A17
  constraint tangent L10 A18
  constraint tangent L5 A19
  constraint tangent L11 A20
  constraint tangent L6 A21
  constraint tangent L3 A22
  constraint tangent L1 A23
  constraint tangent L4 A24
  constraint tangent L15 A25
  constraint tangent A24 L104
  constraint perpendicular L104 L105
  constraint tangent L104 A26
  constraint tangent L105 A26
  constraint coincident L15.end L105
  constraint perpendicular L15 L105
  constraint coincident L14.end L104
  constraint perpendicular L14 L104
  constraint tangent L32 A27
  constraint tangent L33 A28
  constraint tangent L35 A29
  constraint tangent L34 A30
  constraint tangent L49 A31
  constraint tangent L49 A32
  constraint tangent L51 A33
  constraint tangent L50 A34
  constraint tangent L57 A35
  constraint tangent L57 A36
  constraint tangent L59 A37
  constraint tangent L58 A38
  constraint tangent L76 A39
  constraint tangent L78 A40
  constraint tangent L79 A41
  constraint tangent L77 A42
  constraint tangent L54 A43
  constraint tangent L54 A44
  constraint tangent L52 A45
  constraint tangent L53 A46
  constraint tangent L90 A47
  constraint tangent L90 A48
  constraint tangent L91 A48
  constraint tangent L91 A49
  constraint tangent L89 A50
  constraint tangent L100 A51
  constraint tangent L101 A52
  constraint tangent L103 A53
  constraint tangent L102 A54
  constraint tangent L93 A55
  constraint tangent L93 A56
  constraint tangent L95 A57
  constraint tangent L94 A58
  constraint tangent L21 A59
  constraint tangent L20 A60
  constraint tangent L22 A60
  constraint tangent L22 A61
  constraint tangent L23 A62
  constraint tangent L64 A63
  constraint tangent L66 A63
  constraint tangent L64 A64
  constraint tangent L65 A65
  constraint tangent L67 A66
  constraint tangent L98 A67
  constraint tangent L98 A68
  constraint tangent L96 A69
  constraint tangent L97 A70
  constraint tangent L70 A71
  constraint tangent L70 A72
  constraint tangent L68 A73
  constraint tangent L69 A74
  constraint tangent L80 A75
  constraint tangent L80 A76
  constraint tangent L82 A76
  constraint tangent L82 A77
  constraint tangent L83 A77
  constraint tangent L83 A78
  constraint tangent L81 A78
  constraint tangent L29 A79
  constraint tangent L29 A80
  constraint tangent L28 A81
  constraint tangent L30 A82
  constraint tangent L37 A83
  constraint tangent L37 A84
  constraint tangent L36 A84
  constraint tangent L36 A85
  constraint tangent L38 A85
  constraint tangent L38 A86
  constraint tangent L39 A86
  constraint tangent L61 A87
  constraint tangent L61 A88
  constraint tangent L60 A88
  constraint tangent L60 A89
  constraint tangent L62 A90
  constraint tangent L40 A91
  constraint tangent L42 A92
  constraint tangent L43 A93
  constraint tangent L41 A93
  constraint tangent L41 A94
  constraint tangent L40 A94
  constraint tangent L44 A95
  constraint tangent L46 A95
  constraint tangent L46 A96
  constraint tangent L47 A96
  constraint tangent L47 A97
  constraint tangent L45 A97
  constraint tangent L45 A98
  constraint tangent L44 A98
  constraint tangent L74 A99
  constraint tangent L75 A99
  constraint tangent L74 A100
  constraint tangent L72 A101
  constraint tangent L73 A102
  constraint tangent L26 A103
  constraint tangent L27 A103
  constraint tangent L26 A104
  constraint tangent L24 A105
  constraint tangent L25 A106
  constraint tangent L86 A107
  constraint tangent L87 A107
  constraint tangent L86 A108
  constraint tangent L84 A109
  constraint tangent L85 A110
  constraint concentric A26 A132
  constraint concentric A24 A133
  constraint concentric A15 A134
  constraint concentric A14 A135
  constraint tangent A134 L130
  constraint tangent A132 L127
  constraint tangent L127 A133
  constraint tangent L129 A134
  constraint tangent L130 A135
  constraint coincident L114 L131.start
  constraint coincident L127 L131.end
  constraint perpendicular L127 L131
  constraint coincident L113 L132.start
  constraint perpendicular L113 L133
  constraint coincident L113 L133.end
  constraint perpendicular L133 L134
  constraint coincident L114 L135.end
  constraint tangent L136 A138
  constraint tangent L134 A138
  constraint tangent L133 A139
  constraint tangent L134 A139
  constraint tangent L135 A140
  constraint tangent L136 A140
  constraint coincident L114 L137.start
  constraint perpendicular L104 L137
  constraint perpendicular L137 L138
  constraint perpendicular L114 L139
  constraint coincident L114 L139.end
  constraint tangent L137 A141
  constraint tangent L138 A141
  constraint tangent L138 A142
  constraint tangent L139 A142
  constraint concentric A12 A111
  constraint concentric A11 A112
  constraint concentric A10 A113
  constraint concentric A9 A114
  constraint concentric A8 A115
  constraint concentric A7 A116
  constraint concentric A6 A117
  constraint concentric A5 A118
  constraint concentric A26 A119
  constraint concentric A24 A120
  constraint concentric A23 A121
  constraint concentric A22 A122
  constraint concentric A21 A123
  constraint concentric A20 A124
  constraint concentric A19 A125
  constraint concentric A18 A126
  constraint concentric A17 A127
  constraint concentric A16 A128
  constraint concentric A15 A129
  constraint concentric A14 A130
  constraint concentric A13 A131
  constraint tangent L124 A130
  constraint tangent L106 A131
  constraint tangent L123 A129
  constraint tangent A112 L107
  constraint tangent A113 L108
  constraint tangent A117 L112
  constraint tangent A129 L124
  constraint tangent A114 L109
  constraint tangent A115 L110
  constraint tangent A116 L111
  constraint tangent L112 A118
  constraint tangent A120 L115
  constraint tangent L113 A119
  constraint tangent A119 L114
  constraint tangent L114 A120
  constraint tangent A121 L116
  constraint tangent A122 L117
  constraint tangent A126 L121
  constraint tangent A123 L118
  constraint tangent A124 L119
  constraint tangent A125 L120
  constraint tangent A127 L122
  constraint tangent A128 L123
  constraint tangent A130 L125
  constraint tangent A12 L141
  constraint parallel L140 L142
  constraint tangent A111 L143
  constraint tangent L143 A143
  constraint tangent L142 A143
  constraint tangent L140 A144
  constraint tangent L141 A144
  constraint horizontal L144
  constraint tangent L144 A145
  constraint tangent L144 A146
  constraint tangent A135 L146
  constraint tangent A132 L149
  constraint horizontal L150
  constraint horizontal L151
  constraint concentric A8 A147
  constraint concentric A6 A148
  constraint concentric A23 A149
  constraint concentric A21 A150
  constraint horizontal L152
  constraint perpendicular L152 L153
  constraint parallel L152 L154
  constraint parallel L153 L155
  constraint tangent L155 A151
  constraint tangent L154 A151
  constraint tangent L152 A152
  constraint tangent L155 A152
  constraint tangent L152 A153
  constraint tangent L153 A153
  constraint tangent L153 A154
  constraint tangent L154 A154
  constraint horizontal L156
  constraint perpendicular L156 L157
  constraint parallel L156 L158
  constraint parallel L157 L159
  constraint tangent A158 L159
  constraint tangent L158 A158
  constraint tangent A155 L156
  constraint tangent A155 L159
  constraint tangent L156 A156
  constraint tangent A156 L157
  constraint tangent L157 A157
  constraint tangent A157 L158
  constraint horizontal L160
  constraint perpendicular L160 L161
  constraint parallel L160 L162
  constraint parallel L161 L163
  constraint tangent A162 L163
  constraint tangent L162 A162
  constraint tangent A159 L160
  constraint tangent A159 L163
  constraint tangent L160 A160
  constraint tangent A160 L161
  constraint tangent L161 A161
  constraint tangent A161 L162
  constraint horizontal L164
  constraint perpendicular L164 L165
  constraint parallel L164 L166
  constraint parallel L165 L167
  constraint tangent A166 L167
  constraint tangent L166 A166
  constraint tangent A163 L164
  constraint tangent A163 L167
  constraint tangent L164 A164
  constraint tangent A164 L165
  constraint tangent L165 A165
  constraint tangent A165 L166
  constraint horizontal L168
  constraint perpendicular L168 L169
  constraint parallel L168 L170
  constraint parallel L169 L171
  constraint tangent A170 L171
  constraint tangent L170 A170
  constraint tangent A167 L168
  constraint tangent A167 L171
  constraint tangent L168 A168
  constraint tangent A168 L169
  constraint tangent L169 A169
  constraint tangent A169 L170
  constraint horizontal L172
  constraint perpendicular L172 L173
  constraint parallel L172 L174
  constraint parallel L173 L175
  constraint tangent A174 L175
  constraint tangent L174 A174
  constraint tangent A171 L172
  constraint tangent A171 L175
  constraint tangent L172 A172
  constraint tangent A172 L173
  constraint tangent L173 A173
  constraint tangent A173 L174
  constraint horizontal L176
  constraint perpendicular L176 L177
  constraint parallel L176 L178
  constraint parallel L177 L179
  constraint tangent A178 L179
  constraint tangent L178 A178
  constraint tangent A175 L176
  constraint tangent A175 L179
  constraint tangent L176 A176
  constraint tangent A176 L177
  constraint tangent L177 A177
  constraint tangent A177 L178
  constraint horizontal L180
  constraint perpendicular L180 L181
  constraint parallel L180 L182
  constraint parallel L181 L183
  constraint tangent A182 L183
  constraint tangent L182 A182
  constraint tangent A179 L180
  constraint tangent A179 L183
  constraint tangent L180 A180
  constraint tangent A180 L181
  constraint tangent L181 A181
  constraint tangent A181 L182
  constraint horizontal L184
  constraint perpendicular L184 L185
  constraint parallel L184 L186
  constraint parallel L185 L187
  constraint tangent A186 L187
  constraint tangent L186 A186
  constraint tangent A183 L184
  constraint tangent A183 L187
  constraint tangent L184 A184
  constraint tangent A184 L185
  constraint tangent L185 A185
  constraint tangent A185 L186
  constraint horizontal L196
  constraint perpendicular L196 L197
  constraint parallel L196 L198
  constraint parallel L197 L199
  constraint tangent A198 L199
  constraint tangent L198 A198
  constraint tangent A195 L196
  constraint tangent A195 L199
  constraint tangent L196 A196
  constraint tangent A196 L197
  constraint tangent L197 A197
  constraint tangent A197 L198
  constraint horizontal L192
  constraint perpendicular L192 L193
  constraint parallel L192 L194
  constraint parallel L193 L195
  constraint tangent A194 L195
  constraint tangent L194 A194
  constraint tangent A191 L192
  constraint tangent A191 L195
  constraint tangent L192 A192
  constraint tangent A192 L193
  constraint tangent L193 A193
  constraint tangent A193 L194
  constraint horizontal L188
  constraint perpendicular L188 L189
  constraint parallel L188 L190
  constraint parallel L189 L191
  constraint tangent A190 L191
  constraint tangent L190 A190
  constraint tangent A187 L188
  constraint tangent A187 L191
  constraint tangent L188 A188
  constraint tangent A188 L189
  constraint tangent L189 A189
  constraint tangent A189 L190
  constraint horizontal L208
  constraint perpendicular L208 L209
  constraint parallel L208 L210
  constraint parallel L209 L211
  constraint tangent A210 L211
  constraint tangent L210 A210
  constraint tangent A207 L208
  constraint tangent A207 L211
  constraint tangent L208 A208
  constraint tangent A208 L209
  constraint tangent L209 A209
  constraint tangent A209 L210
  constraint horizontal L204
  constraint perpendicular L204 L205
  constraint parallel L204 L206
  constraint parallel L205 L207
  constraint tangent A206 L207
  constraint tangent L206 A206
  constraint tangent A203 L204
  constraint tangent A203 L207
  constraint tangent L204 A204
  constraint tangent A204 L205
  constraint tangent L205 A205
  constraint tangent A205 L206
  constraint horizontal L200
  constraint perpendicular L200 L201
  constraint parallel L200 L202
  constraint parallel L201 L203
  constraint tangent A202 L203
  constraint tangent L202 A202
  constraint tangent A199 L200
  constraint tangent A199 L203
  constraint tangent L200 A200
  constraint tangent A200 L201
  constraint tangent L201 A201
  constraint tangent A201 L202
  constraint horizontal L212
  constraint perpendicular L212 L213
  constraint parallel L212 L214
  constraint parallel L213 L215
  constraint tangent A214 L215
  constraint tangent L214 A214
  constraint tangent A211 L212
  constraint tangent A211 L215
  constraint tangent L212 A212
  constraint tangent A212 L213
  constraint tangent L213 A213
  constraint tangent A213 L214
  constraint horizontal L228
  constraint perpendicular L228 L229
  constraint parallel L228 L230
  constraint parallel L229 L231
  constraint tangent A230 L231
  constraint tangent L230 A230
  constraint tangent A227 L228
  constraint tangent A227 L231
  constraint tangent L228 A228
  constraint tangent A228 L229
  constraint tangent L229 A229
  constraint tangent A229 L230
  constraint horizontal L224
  constraint perpendicular L224 L225
  constraint parallel L224 L226
  constraint parallel L225 L227
  constraint tangent A226 L227
  constraint tangent L226 A226
  constraint tangent A223 L224
  constraint tangent A223 L227
  constraint tangent L224 A224
  constraint tangent A224 L225
  constraint tangent L225 A225
  constraint tangent A225 L226
  constraint horizontal L220
  constraint perpendicular L220 L221
  constraint parallel L220 L222
  constraint parallel L221 L223
  constraint tangent A222 L223
  constraint tangent L222 A222
  constraint tangent A219 L220
  constraint tangent A219 L223
  constraint tangent L220 A220
  constraint tangent A220 L221
  constraint tangent L221 A221
  constraint tangent A221 L222
  constraint horizontal L216
  constraint perpendicular L216 L217
  constraint parallel L216 L218
  constraint parallel L217 L219
  constraint tangent A218 L219
  constraint tangent L218 A218
  constraint tangent A215 L216
  constraint tangent A215 L219
  constraint tangent L216 A216
  constraint tangent A216 L217
  constraint tangent L217 A217